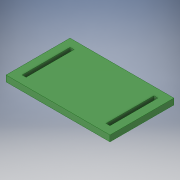
# Autodesk Inventor part: 5x3holder
Saved by Autodesk Inventor 2019 (Build 230136000, 136)
## iProperties
Created: 2019-02-19
Part Number: 5x3holder
Material: PET Plastic
Document SubType Name: Modeling
Designer: jmc
Density: 1.541 g/cm^3
Appearance: Smooth - Dark Forest Green
Author: jmc
Autodesk Inventor part; units mm, degrees
ref_plane "YZ Plane" through (0, 0, 0) normal (1, 0, 0) x (0, 1, 0)
ref_plane "XZ Plane" through (0, 0, 0) normal (0, 1, 0) x (-1, 0, 0)
ref_plane "XY Plane" through (0, 0, 0) normal (0, 0, 1) x (1, 0, 0)
sketch "Sketch1" plane through (0, 0, 0) normal (0, 1, 0) x (-1, 0, 0)
  line L0 (26, 16) -> (-26, 16)
  line L1 (-26, 16) -> (-26, -16)
  line L2 (-26, -16) -> (26, -16)
  line L3 (26, -16) -> (26, 16)
  line L4 (26, 16) -> (-26, -16) construction
  line L5 (-26, 16) -> (26, -16) construction
  point P0 (0, 0)
  dimension "d0" = 52
  dimension "d1" = 32
  constraints: 12 end point, 2 midpoint, 2 parallel, 1 horizontal, 1 perpendicular
  measures "d0" distance of L2.end L1.end
  measures "d1" distance of L1.end L0.end
extrude "Extrusion1" add sketch "Sketch1" along normal blind 2
sketch "Sketch2" plane through (0, 0, 0) normal (0, -1, 0) x (1, 0, 0)
  point P0 (0, 0)
sketch "Sketch3" plane through (0, 0, 0) normal (0, -1, 0) x (1, 0, 0)
  line L0 (-26, 16) -> (26, 16) projected
  line L1 (-26, -16) -> (-26, 16) projected
  line L2 (26, -16) -> (-26, -16) projected
  line L3 (26, 16) -> (26, -16) projected
  line L4 (24, 14) -> (-24, 14)
  line L5 (-24, 14) -> (-24, -14)
  line L6 (-24, -14) -> (24, -14)
  line L7 (24, -14) -> (24, 14)
  point P0 (0, 0)
  dimension "d4" = 2
  constraints: 8 end point, 3 other
  measures "d4" distance between parallel lines of L0 L4
extrude "Extrusion2" add sketch "Sketch3" along normal blind 1
sketch "Sketch4" plane through (0, 0, 0) normal (0, -1, 0) x (1, 0, 0)
  point P0 (0, 0)
sketch "Sketch5" plane through (0, 2, 0) normal (0, 1, 0) x (1, 0, 0)
  line L0 (-22, 12) -> (-20, 12)
  line L1 (-20, 12) -> (-20, -12)
  line L2 (-20, -12) -> (-22, -12)
  line L3 (-22, -12) -> (-22, 12)
  line L4 (-26, 16) -> (-26, -16) projected
  line L5 (26, 16) -> (-26, 16) projected
  line L6 (-26, -16) -> (26, -16) projected
  point P0 (0, 0)
  dimension "d7" = 2
  dimension "d8" = 4
  dimension "d9" = 4
  dimension "d10" = 4
  constraints: 8 end point, 2 parallel, 1 horizontal, 1 perpendicular
  measures "d7" distance between parallel lines of L1 L3
  measures "d8" distance between parallel lines of L4 L3
  measures "d9" distance between parallel lines of L5 L0
  measures "d10" distance between parallel lines of L6 L2
extrude "Extrusion3" cut sketch "Sketch5" against normal through all
mirror "Mirror1" about plane through (0, 0, 0) normal (1, 0, 0) of "Extrusion3"
body "Solid1"
